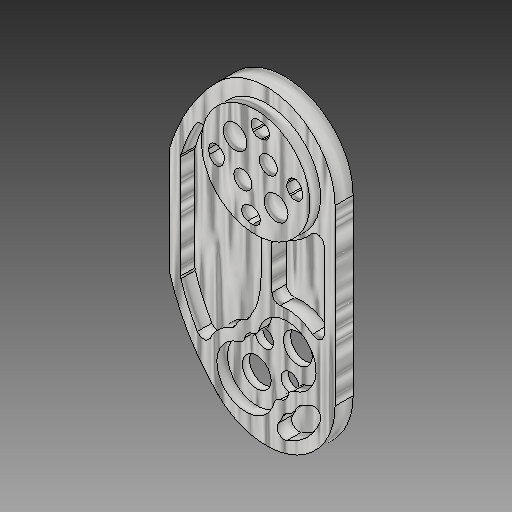
# Autodesk Inventor part: 新型３クランク
Saved by Autodesk Inventor 2019 (Build 230136000, 136)
## iProperties
Created: 2019-04-13
Part Number: 新型３クランク
Material: アルミニウム 7075
Document SubType Name: Modeling
Designer: tanjihayato
Density: 2.81 g/cm^3
Appearance: サテン - ブラシ仕上げ 重厚
Mass: 3.99356 g
Surface Area: 24.6385 cm^2
Volume: 1.42119 cm^3
Author: tanjihayato
Autodesk Inventor part; units mm, degrees
ref_plane "YZ Plane" through (0, 0, 0) normal (1, 0, 0) x (0, 1, 0)
ref_plane "XZ Plane" through (0, 0, 0) normal (0, 1, 0) x (-1, 0, 0)
ref_plane "XY Plane" through (0, 0, 0) normal (0, 0, 1) x (1, 0, 0)
sketch "スケッチ1" plane through (0, 0, 0) normal (0, 0, 1) x (1, 0, 0)
  circle A0 centre (-9.17471, -9.17471) radius 2
  circle A1 centre (-14.86692, -14.86692) radius 2
  circle A2 centre (-13.788582, -10.253048) radius 1.25
  circle A3 centre (-10.253048, -13.788582) radius 1.25
  arc A4 (-8.249894, -13.092023) -> (-9.012536, -13.942297) centre (-8.020125, -14.065269) ccw
  arc A5 (-10.099334, -15.029095) -> (-9.012536, -13.942297) centre (-10.253048, -13.788582) ccw
  arc A6 (-10.099334, -15.029095) -> (-10.949607, -15.791737) centre (-9.976362, -16.021505) ccw
  arc A7 (-15.791737, -10.949607) -> (-10.949607, -15.791737) centre (-14.86692, -14.86692) ccw
  arc A8 (-15.791737, -10.949607) -> (-15.029095, -10.099334) centre (-16.021505, -9.976362) ccw
  arc A9 (-13.942297, -9.012536) -> (-15.029095, -10.099334) centre (-13.788582, -10.253048) ccw
  arc A10 (-13.942297, -9.012536) -> (-13.092023, -8.249894) centre (-14.065269, -8.020125) ccw
  arc A11 (-8.249894, -13.092023) -> (-13.092023, -8.249894) centre (-9.17471, -9.17471) ccw
  circle A12 centre (-10.253048, 13.788582) radius 1.25
  circle A13 centre (-13.788582, 10.253048) radius 1.25
  circle A14 centre (-9.17471, 9.17471) radius 1.65
  circle A15 centre (-14.86692, 14.86692) radius 1.65
  line L0 (-14.86692, 14.86692) -> (-9.17471, 9.17471)
  line L1 (-10.253048, 13.788582) -> (-13.788582, 10.253048)
  line L2 (-9.17471, -9.17471) -> (-14.86692, -14.86692)
  line L3 (-13.788582, -10.253048) -> (-10.253048, -13.788582)
  circle A16 centre (-12.020815, 12.020815) radius 9.5
  circle A17 centre (-12.020815, -12.020815) radius 9.5
  arc A18 (-18.73833, 18.73833) -> (-18.73833, -18.73833) centre (0, 0) ccw
  arc A19 (-5.303301, -18.73833) -> (-5.303301, 18.73833) centre (-24.041631, 0) ccw
  point P0 (0, 0)
  dimension "d0" = 19
  dimension "d1" = 19
  dimension "d2" = 17
  dimension "d3" = 17
  dimension "d101" = 3.3
  dimension "d102" = 3.3
  constraints: 32 centre point, 24 point on circle, 8 end point, 4 tangent, 2 midpoint, 2 perpendicular, 1 coincident, 1 parallel, 2 other
  measures "d0" diameter of A16
  measures "d1" diameter of A17
  measures "d2" distance of A16.centre A18.centre
  measures "d3" distance of A16.centre A19.centre
  measures "d101" diameter of A14
  measures "d102" diameter of A15
sketch "スケッチ2" plane through (0, 0, 0) normal (0, 0, 1) x (1, 0, 0)
  circle A0 centre (-12.020815, 12.020815) radius 9.5
  arc A1 (-18.73833, 18.73833) -> (-18.73833, -18.73833) centre (0, 0) ccw
  circle A2 centre (-14.86692, 14.86692) radius 1.65
  circle A3 centre (-10.253048, 13.788582) radius 1.25
  circle A4 centre (-13.788582, 10.253048) radius 1.25
  circle A5 centre (-9.17471, 9.17471) radius 1.65
  circle A6 centre (-12.020815, -12.020815) radius 9.5
  arc A7 (-8.249894, -13.092023) -> (-13.092023, -8.249894) centre (-9.17471, -9.17471) ccw
  circle A8 centre (-9.17471, -9.17471) radius 2
  circle A9 centre (-13.788582, -10.253048) radius 1.25
  arc A10 (-13.942297, -9.012536) -> (-13.092023, -8.249894) centre (-14.065269, -8.020125) ccw
  arc A11 (-15.791737, -10.949607) -> (-15.029095, -10.099334) centre (-16.021505, -9.976362) ccw
  arc A12 (-15.791737, -10.949607) -> (-10.949607, -15.791737) centre (-14.86692, -14.86692) ccw
  circle A13 centre (-14.86692, -14.86692) radius 2
  circle A14 centre (-10.253048, -13.788582) radius 1.25
  arc A15 (-10.099334, -15.029095) -> (-10.949607, -15.791737) centre (-9.976362, -16.021505) ccw
  arc A16 (-10.099334, -15.029095) -> (-9.012536, -13.942297) centre (-10.253048, -13.788582) ccw
  arc A17 (-8.249894, -13.092023) -> (-9.012536, -13.942297) centre (-8.020125, -14.065269) ccw
  arc A18 (-7.629655, -14.427179) -> (-14.427179, -7.629655) centre (-9.17471, -9.17471) ccw
  arc A19 (-9.614451, -16.411976) -> (-7.629655, -14.427179) centre (-10.253048, -13.788582) ccw
  arc A20 (-16.411976, -9.614451) -> (-9.614451, -16.411976) centre (-14.86692, -14.86692) ccw
  arc A21 (-14.427179, -7.629655) -> (-16.411976, -9.614451) centre (-13.788582, -10.253048) ccw
  arc A22 (-11.918863, 15.976632) -> (-15.976632, 11.918863) centre (-14.86692, 14.86692) ccw
  arc A23 (-8.064999, 12.122767) -> (-11.918863, 15.976632) centre (-10.253048, 13.788582) ccw
  arc A24 (-15.976632, 11.918863) -> (-12.122767, 8.064999) centre (-13.788582, 10.253048) ccw
  arc A25 (-12.122767, 8.064999) -> (-8.064999, 12.122767) centre (-9.17471, 9.17471) ccw
  circle A26 centre (-12.020815, -12.020815) radius 8
  line L0 (-25.41653, 7.5) -> (-25.41653, -7.5)
  line L1 (-23.91653, 7.280082) -> (-23.91653, -7.280082)
  arc A27 (-21.491034, 12.772449) -> (-23.91653, 7.280082) centre (0, 0) ccw
  arc A28 (-23.91653, -7.280082) -> (-21.491034, -12.772449) centre (0, 0) ccw
  line L2 (-2.520815, 12.020815) -> (-2.520815, -12.020815)
  line L3 (-4.020815, 6.89734) -> (-4.020815, -6.89734)
  circle A29 centre (-12.020815, 12.020815) radius 7.5
  line L4 (-13.788582, -10.253048) -> (-4.046147, -19.995484) construction
  line L5 (-13.788582, 10.253048) -> (-4.086909, 19.954722) construction
  line L6 (-12.770815, 2.550467) -> (-12.770815, -2.550467)
  line L7 (-11.270815, 2.550467) -> (-11.270815, -2.550467)
  point P0 (0, 0)
  point P1 (-5.303301, -18.73833)
  point P2 (-5.303301, 18.73833)
  dimension "d5" = 1.45
  dimension "d7" = 1.45
  dimension "d12" = 1.5
  dimension "d13" = 1.5
  dimension "d14" = 1.5
  dimension "d15" = 1.5
  dimension "d19" = 1.5
  dimension "d20" = 15
  dimension "d21" = 1.5
  dimension "d22" = 1.5
  dimension "d23" = 1.5
  dimension "d24" = 1.5
  dimension "d29" = 15
  dimension "d33" = 1.5
  dimension "d34" = 0.75
  constraints: 22 point on circle, 16 end point, 12 centre point, 6 vertical, 2 point on line, 1 coincident, 1 parallel, 14 other
  measures "d5" radial gap between concentric circles of A16 A19
  measures "d7" radial gap between concentric circles of A9 A21
  measures "d12" radial gap between concentric circles of A3 A23
  measures "d13" radial gap between concentric circles of A2 A22
  measures "d14" radial gap between concentric circles of A24 A4
  measures "d15" radial gap between concentric circles of A25 A5
  measures "d20" distance of L0.start L0.end
  measures "d21" distance between parallel lines of L1 L0
  measures "d22" radial gap between concentric circles of A1 A27
  measures "d23" radial gap between concentric circles of A1 A28
  measures "d24" distance between parallel lines of L3 L2
  measures "d29" diameter of A29
  measures "d33" distance between parallel lines of L6 L7
  measures "d34" distance from line of point (-12.021, 12.021) L7
extrude "押し出し4" add sketch "スケッチ2" along normal blind 4 contours A23 A25 A24 A22 | A29
extrude "押し出し5" add sketch "スケッチ2" along normal blind 2.5 contours A0 | L2 A6 L3 A0 | A0 A27 L1 A28 A6 A1 L0 | A6 A20 A26 A18 | L7 A6 L6 A0 | A6 A18 A26 A20 | A20 A26 A12 | A18 A26 A7 | A20 A21 A18 A26 A7 A10 A9 A11 A12 | A26 A12 A15 A14 A17 A7 A18 A19 A20
extrude "押し出し6" add sketch "スケッチ2" along normal blind 1 contours A26 A12 | A12 A11 A9 A10 A7 A26 A17 A14 A15 | A26 A7
extrude "押し出し7" add sketch "スケッチ2" along normal blind 0.5 contours L3 A6 L7 A0 | A0 L6 A6 A28 L1 A27 | A26 A18 A21 A20 | A20 A21 A18 A26 A7 A10 A9 A11 A12 | A26 A12 A15 A14 A17 A7 A18 A19 A20 | A20 A19 A18 A26 | A12 A11 A9 A10 A7 A26 A17 A14 A15
extrude "押し出し8" add sketch "スケッチ2" along normal blind 1 contours A3 | A4
sketch "スケッチ3" plane through (-12.020815, 12.020815, 4) normal (0, 0, 1) x (1, 0, 0)
  circle A0 centre (2.846105, -2.846105) radius 1.65
  circle A1 centre (-2.846105, 2.846105) radius 1.65
  circle A2 centre (-1.767767, -1.767767) radius 1.25
  circle A3 centre (1.767767, 1.767767) radius 1.25
  circle A4 centre (0, 0) radius 7.5
  arc A5 (9.5, 0) -> (-6.717514, 6.717514) centre (0, 0) ccw
  circle A6 centre (-2.846105, 2.846105) radius 3.15
  circle A7 centre (2.846105, -2.846105) radius 3.15
  line L0 (-1.767767, -1.767767) -> (9.834677, 9.834677) construction
  arc A8 (-0.156324, 7.998473) -> (1.213798, 4.461392) centre (9.834677, 9.834677) ccw
  arc A9 (4.461392, 1.213798) -> (7.998473, -0.156324) centre (9.834677, 9.834677) ccw
  arc A10 (4.461392, 1.213798) -> (1.213798, 4.461392) centre (1.767767, 1.767767) ccw
  arc A11 (0.096916, 3.969104) -> (3.969104, 0.096916) centre (1.767767, 1.767767) ccw
  line L1 (9.5, -24.041631) -> (9.5, 0)
  arc A12 (-9.470219, 0.751633) -> (-0.75, -9.470348) centre (0, 0) ccw
  arc A13 (0.156324, -7.998473) -> (-1.213798, -4.461392) centre (-9.834677, -9.834677) ccw
  arc A14 (-4.461392, -1.213798) -> (-7.998473, 0.156324) centre (-9.834677, -9.834677) ccw
  arc A15 (-4.461392, -1.213798) -> (-1.213798, -4.461392) centre (-1.767767, -1.767767) ccw
  arc A16 (-0.096916, -3.969104) -> (-3.969104, -0.096916) centre (-1.767767, -1.767767) ccw
  circle A17 centre (0, 0) radius 8
  point P0 (12.020815, -12.020815)
  point P1 (-0.051687, 7.499822)
  point P2 (7.499822, -0.051687)
  point P3 (0.051687, -7.499822)
  point P4 (-7.499822, 0.051687)
  dimension "d46" = 1.5
  dimension "d47" = 1.5
  dimension "d53" = 16
  constraints: 32 point on circle, 11 centre point, 2 end point, 2 point on line, 1 coincident, 4 other
  measures "d46" radial gap between concentric circles of A1 A6
  measures "d47" radial gap between concentric circles of A0 A7
  measures "d53" diameter of A17
extrude "押し出し11" cut sketch "スケッチ3" against normal blind 3.5 contours A4 A9 A10 A8 | A4 A8 A17 A9 | A14 A15 A13 A4 | A4 A13 A17 A14
fillet "フィレット1" radius 1 26 edges at (-4.0223, 11.8645, 1.5) (-11.8645, 4.0223, 1.5) (-20.0193, 12.1771, 1.5) (-12.1771, 20.0193, 1.5) (-13.2346, 7.5594, 2.25) (-16.4822, 10.807, 2.25) (-10.807, 16.4822, 2.25) (-7.5594, 13.2346, 2.25) (-12.7708, 2.5505, 1.5) (-21.491, 12.7724, 1.5) (-21.491, -12.7724, 1.5) (-23.9165, 7.2801, 1.5) (-23.9165, -7.2801, 1.5) (-12.7708, -2.5505, 1.5) (-11.2708, -2.5505, 1.5) (-11.2708, 2.5505, 1.5) (-4.0208, 6.8973, 1.5) (-4.0208, -6.8973, 1.5) (-4.0684, -11.1498, 1.5) (-12.8918, -19.9733, 1.5) (-9.6145, -16.412, 1.5) (-7.6297, -14.4272, 1.5) (-14.4272, -7.6297, 1.5) (-16.412, -9.6145, 1.5) (-19.9733, -12.8918, 1.5) (-11.1498, -4.0684, 1.5)
sketch "スケッチ5" plane through (0, 0, 2.5) normal (0, 0, 1) x (1, 0, 0)
  arc A0 (-9.205581, -19.509103) -> (-4.532527, -14.83605) centre (-12.020815, -12.020815) ccw
  arc A1 (-10.377475, -18.000689) -> (-9.205581, -19.509103) centre (-9.557485, -18.573067) ccw
  arc A2 (-10.377475, -18.000689) -> (-9.760725, -16.842368) centre (-14.86692, -14.86692) ccw
  arc A3 (-9.213211, -16.280316) -> (-9.760725, -16.842368) centre (-8.828087, -17.203181) ccw
  arc A4 (-9.213211, -16.280316) -> (-7.761314, -14.828419) centre (-10.253048, -13.788582) ccw
  arc A5 (-7.199262, -14.280906) -> (-7.761314, -14.828419) centre (-6.83845, -15.213544) ccw
  arc A6 (-7.199262, -14.280906) -> (-6.040941, -13.664155) centre (-9.17471, -9.17471) ccw
  arc A7 (-4.532527, -14.83605) -> (-6.040941, -13.664155) centre (-5.468563, -14.484145) ccw
  arc A8 (-14.828419, -7.761314) -> (-14.280906, -7.199262) centre (-15.213544, -6.83845) ccw
  arc A9 (-14.828419, -7.761314) -> (-16.280316, -9.213211) centre (-13.788582, -10.253048) ccw
  arc A10 (-16.842368, -9.760725) -> (-16.280316, -9.213211) centre (-17.203181, -8.828087) ccw
  arc A11 (-16.842368, -9.760725) -> (-18.000689, -10.377475) centre (-14.86692, -14.86692) ccw
  arc A12 (-19.509103, -9.205581) -> (-18.000689, -10.377475) centre (-18.573067, -9.557485) ccw
  arc A13 (-14.83605, -4.532527) -> (-19.509103, -9.205581) centre (-12.020815, -12.020815) ccw
  arc A14 (-13.664155, -6.040941) -> (-14.83605, -4.532527) centre (-14.484145, -5.468563) ccw
  arc A15 (-13.664155, -6.040941) -> (-14.280906, -7.199262) centre (-9.17471, -9.17471) ccw
  arc A16 (-11.671378, 19.51267) -> (-19.51267, 11.671378) centre (-12.020815, 12.020815) ccw
  arc A17 (-10.697307, 19.910576) -> (-11.671378, 19.51267) centre (-10.862746, 18.924356) ccw
  arc A18 (-4.131054, 13.344324) -> (-10.697307, 19.910576) centre (-12.020815, 12.020815) ccw
  arc A19 (-4.52896, 12.370253) -> (-4.131054, 13.344324) centre (-5.117275, 13.178885) ccw
  arc A20 (-12.370253, 4.52896) -> (-4.52896, 12.370253) centre (-12.020815, 12.020815) ccw
  arc A21 (-13.344324, 4.131054) -> (-12.370253, 4.52896) centre (-13.178885, 5.117275) ccw
  arc A22 (-19.910576, 10.697307) -> (-13.344324, 4.131054) centre (-12.020815, 12.020815) ccw
  arc A23 (-19.51267, 11.671378) -> (-19.910576, 10.697307) centre (-18.924356, 10.862746) ccw
  arc A24 (-8.249894, -13.092023) -> (-13.092023, -8.249894) centre (-9.17471, -9.17471) ccw
  arc A25 (-8.249894, -13.092023) -> (-9.012536, -13.942297) centre (-8.020125, -14.065269) ccw
  arc A26 (-10.099334, -15.029095) -> (-9.012536, -13.942297) centre (-10.253048, -13.788582) ccw
  arc A27 (-10.099334, -15.029095) -> (-10.949607, -15.791737) centre (-9.976362, -16.021505) ccw
  arc A28 (-15.791737, -10.949607) -> (-10.949607, -15.791737) centre (-14.86692, -14.86692) ccw
  arc A29 (-15.791737, -10.949607) -> (-15.029095, -10.099334) centre (-16.021505, -9.976362) ccw
  arc A30 (-13.942297, -9.012536) -> (-15.029095, -10.099334) centre (-13.788582, -10.253048) ccw
  arc A31 (-13.942297, -9.012536) -> (-13.092023, -8.249894) centre (-14.065269, -8.020125) ccw
  line L0 (-12.770815, 1.667676) -> (-12.770815, -1.667676)
  arc A32 (-13.604149, -2.653689) -> (-12.770815, -1.667676) centre (-13.770815, -1.667676) ccw
  arc A33 (-13.604149, -2.653689) -> (-21.183069, -9.510218) centre (-12.020815, -12.020815) ccw
  arc A34 (-23.07033, -9.631192) -> (-21.183069, -9.510218) centre (-22.147517, -9.245944) ccw
  arc A35 (-23.871385, -7.426773) -> (-23.07033, -9.631192) centre (0, 0) ccw
  arc A36 (-23.91653, -7.129702) -> (-23.871385, -7.426773) centre (-22.91653, -7.129702) ccw
  line L1 (-23.91653, -7.129702) -> (-23.91653, 7.129702)
  arc A37 (-23.871385, 7.426773) -> (-23.91653, 7.129702) centre (-22.91653, 7.129702) ccw
  arc A38 (-23.07033, 9.631192) -> (-23.871385, 7.426773) centre (0, 0) ccw
  arc A39 (-21.183069, 9.510218) -> (-23.07033, 9.631192) centre (-22.147517, 9.245944) ccw
  arc A40 (-21.183069, 9.510218) -> (-13.604149, 2.653689) centre (-12.020815, 12.020815) ccw
  arc A41 (-12.770815, 1.667676) -> (-13.604149, 2.653689) centre (-13.770815, 1.667676) ccw
  line L2 (-4.020815, 4.194577) -> (-4.020815, -4.194577)
  arc A42 (-5.687482, -4.939933) -> (-4.020815, -4.194577) centre (-5.020815, -4.194577) ccw
  arc A43 (-5.687482, -4.939933) -> (-10.437482, -2.653689) centre (-12.020815, -12.020815) ccw
  arc A44 (-11.270815, -1.667676) -> (-10.437482, -2.653689) centre (-10.270815, -1.667676) ccw
  line L3 (-11.270815, -1.667676) -> (-11.270815, 1.667676)
  arc A45 (-10.437482, 2.653689) -> (-11.270815, 1.667676) centre (-10.270815, 1.667676) ccw
  arc A46 (-10.437482, 2.653689) -> (-5.687482, 4.939933) centre (-12.020815, 12.020815) ccw
  arc A47 (-4.020815, 4.194577) -> (-5.687482, 4.939933) centre (-5.020815, 4.194577) ccw
  arc A48 (-2.520815, 12.020815) -> (-18.73833, 18.73833) centre (-12.020815, 12.020815) ccw
  arc A49 (-18.73833, 18.73833) -> (-25.41653, 7.5) centre (0, 0) ccw
  line L4 (-25.41653, 7.5) -> (-25.41653, -7.5)
  arc A50 (-25.41653, -7.5) -> (-18.73833, -18.73833) centre (0, 0) ccw
  arc A51 (-18.73833, -18.73833) -> (-2.520815, -12.020815) centre (-12.020815, -12.020815) ccw
  line L5 (-2.520815, -12.020815) -> (-2.520815, 12.020815)
  arc A52 (-19.509103, -9.205581) -> (-18.000689, -10.377475) centre (-18.573067, -9.557485) ccw
  arc A53 (-18.000689, -10.377475) -> (-20.332512, -14.546097) centre (-14.86692, -14.86692) ccw
  arc A54 (-23.07033, -9.631192) -> (-20.332512, -14.546097) centre (0, 0) ccw
  arc A55 (-13.552192, -5.831142) -> (-12.770815, -1.667676) centre (-24.253751, -1.667676) ccw
  point P0 (0, 0)
  constraints: 7 point on circle, 3 centre point, 2 tangent
extrude "押し出し12" cut sketch "スケッチ5" against normal blind 2 contours A14 A13 A12 A53 A54 A34 A33 A32 A55
fillet "フィレット2" radius 1 1 edges at (-20.3325, -14.5461, 1.5)
sketch "スケッチ6" plane through (0, 0, 2.5) normal (0, 0, 1) x (1, 0, 0)
  arc A0 (-2.520815, 12.020815) -> (-18.73833, 18.73833) centre (-12.020815, 12.020815) ccw
  arc A1 (-18.73833, 18.73833) -> (-25.41653, 7.5) centre (0, 0) ccw
  line L0 (-25.41653, 7.5) -> (-25.41653, -7.5)
  arc A2 (-25.41653, -7.5) -> (-18.73833, -18.73833) centre (0, 0) ccw
  arc A3 (-18.73833, -18.73833) -> (-2.520815, -12.020815) centre (-12.020815, -12.020815) ccw
  line L1 (-2.520815, -12.020815) -> (-2.520815, 12.020815)
  line L2 (-4.020815, 4.194577) -> (-4.020815, -4.194577)
  arc A4 (-5.687482, -4.939933) -> (-4.020815, -4.194577) centre (-5.020815, -4.194577) ccw
  arc A5 (-5.687482, -4.939933) -> (-10.437482, -2.653689) centre (-12.020815, -12.020815) ccw
  arc A6 (-11.270815, -1.667676) -> (-10.437482, -2.653689) centre (-10.270815, -1.667676) ccw
  line L3 (-11.270815, -1.667676) -> (-11.270815, 1.667676)
  arc A7 (-10.437482, 2.653689) -> (-11.270815, 1.667676) centre (-10.270815, 1.667676) ccw
  arc A8 (-10.437482, 2.653689) -> (-5.687482, 4.939933) centre (-12.020815, 12.020815) ccw
  arc A9 (-4.020815, 4.194577) -> (-5.687482, 4.939933) centre (-5.020815, 4.194577) ccw
  arc A10 (-8.249894, -13.092023) -> (-13.092023, -8.249894) centre (-9.17471, -9.17471) ccw
  arc A11 (-8.249894, -13.092023) -> (-9.012536, -13.942297) centre (-8.020125, -14.065269) ccw
  arc A12 (-10.099334, -15.029095) -> (-9.012536, -13.942297) centre (-10.253048, -13.788582) ccw
  arc A13 (-10.099334, -15.029095) -> (-10.949607, -15.791737) centre (-9.976362, -16.021505) ccw
  arc A14 (-15.791737, -10.949607) -> (-10.949607, -15.791737) centre (-14.86692, -14.86692) ccw
  arc A15 (-15.791737, -10.949607) -> (-15.029095, -10.099334) centre (-16.021505, -9.976362) ccw
  arc A16 (-13.942297, -9.012536) -> (-15.029095, -10.099334) centre (-13.788582, -10.253048) ccw
  arc A17 (-13.942297, -9.012536) -> (-13.092023, -8.249894) centre (-14.065269, -8.020125) ccw
  arc A18 (-19.910576, 10.697307) -> (-13.344324, 4.131054) centre (-12.020815, 12.020815) ccw
  arc A19 (-19.51267, 11.671378) -> (-19.910576, 10.697307) centre (-18.924356, 10.862746) ccw
  arc A20 (-11.671378, 19.51267) -> (-19.51267, 11.671378) centre (-12.020815, 12.020815) ccw
  arc A21 (-10.697307, 19.910576) -> (-11.671378, 19.51267) centre (-10.862746, 18.924356) ccw
  arc A22 (-4.131054, 13.344324) -> (-10.697307, 19.910576) centre (-12.020815, 12.020815) ccw
  arc A23 (-4.52896, 12.370253) -> (-4.131054, 13.344324) centre (-5.117275, 13.178885) ccw
  arc A24 (-12.370253, 4.52896) -> (-4.52896, 12.370253) centre (-12.020815, 12.020815) ccw
  arc A25 (-13.344324, 4.131054) -> (-12.370253, 4.52896) centre (-13.178885, 5.117275) ccw
  arc A26 (-13.552192, -5.831142) -> (-12.770815, -1.667676) centre (-24.253751, -1.667676) ccw
  arc A27 (-13.664155, -6.040941) -> (-13.552192, -5.831142) centre (-14.484145, -5.468563) ccw
  arc A28 (-13.664155, -6.040941) -> (-14.280906, -7.199262) centre (-9.17471, -9.17471) ccw
  arc A29 (-14.828419, -7.761314) -> (-14.280906, -7.199262) centre (-15.213544, -6.83845) ccw
  arc A30 (-14.828419, -7.761314) -> (-16.280316, -9.213211) centre (-13.788582, -10.253048) ccw
  arc A31 (-16.842368, -9.760725) -> (-16.280316, -9.213211) centre (-17.203181, -8.828087) ccw
  arc A32 (-16.842368, -9.760725) -> (-19.818975, -12.531802) centre (-14.86692, -14.86692) ccw
  arc A33 (-21.586938, -12.609684) -> (-19.818975, -12.531802) centre (-20.72346, -12.105297) ccw
  arc A34 (-23.871385, -7.426773) -> (-21.586938, -12.609684) centre (0, 0) ccw
  arc A35 (-23.91653, -7.129702) -> (-23.871385, -7.426773) centre (-22.91653, -7.129702) ccw
  line L4 (-23.91653, -7.129702) -> (-23.91653, 7.129702)
  arc A36 (-23.871385, 7.426773) -> (-23.91653, 7.129702) centre (-22.91653, 7.129702) ccw
  arc A37 (-23.07033, 9.631192) -> (-23.871385, 7.426773) centre (0, 0) ccw
  arc A38 (-21.183069, 9.510218) -> (-23.07033, 9.631192) centre (-22.147517, 9.245944) ccw
  arc A39 (-21.183069, 9.510218) -> (-13.604149, 2.653689) centre (-12.020815, 12.020815) ccw
  arc A40 (-12.770815, 1.667676) -> (-13.604149, 2.653689) centre (-13.770815, 1.667676) ccw
  line L5 (-12.770815, 1.667676) -> (-12.770815, -1.667676)
  arc A41 (-9.205581, -19.509103) -> (-4.532527, -14.83605) centre (-12.020815, -12.020815) ccw
  arc A42 (-10.377475, -18.000689) -> (-9.205581, -19.509103) centre (-9.557485, -18.573067) ccw
  arc A43 (-10.377475, -18.000689) -> (-9.760725, -16.842368) centre (-14.86692, -14.86692) ccw
  arc A44 (-9.213211, -16.280316) -> (-9.760725, -16.842368) centre (-8.828087, -17.203181) ccw
  arc A45 (-9.213211, -16.280316) -> (-7.761314, -14.828419) centre (-10.253048, -13.788582) ccw
  arc A46 (-7.199262, -14.280906) -> (-7.761314, -14.828419) centre (-6.83845, -15.213544) ccw
  arc A47 (-7.199262, -14.280906) -> (-6.040941, -13.664155) centre (-9.17471, -9.17471) ccw
  arc A48 (-4.532527, -14.83605) -> (-6.040941, -13.664155) centre (-5.468563, -14.484145) ccw
  arc A49 (-5.662343, -4.974841) -> (-11.270815, -4.116848) centre (-9.17471, -9.17471) ccw
  line L6 (-11.270815, -1.667676) -> (-11.270815, -4.116848)
  arc A50 (-5.662343, -4.974841) -> (-4.020815, -4.207742) centre (-5.020815, -4.207742) ccw
  line L7 (-4.020815, 4.194577) -> (-4.020815, -4.194577)
  line L8 (-4.020815, -4.194577) -> (-4.020815, -4.207742)
  point P0 (0, 0)
  dimension "d60" = 2
  dimension "d61" = 1.45
  constraints: 4 end point, 4 point on circle, 2 centre point, 2 tangent, 2 vertical
  measures "d60" diameter of A50
  measures "d61" radial gap between concentric circles of A49 A10
extrude "押し出し13" cut sketch "スケッチ6" against normal blind 2 contours A50 A49 L6 A6 A5 A4
fillet "フィレット3" radius 1 1 edges at (-11.2708, -4.1168, 1.5)
sketch "スケッチ7" plane through (0, 0, 4) normal (0, 0, 1) x (1, 0, 0)
  arc A0 (-12.231485, 5.437326) -> (-12.896473, 6.974428) centre (-21.855492, 2.186138) ccw
  arc A1 (-12.370253, 4.52896) -> (-12.231485, 5.437326) centre (-13.178885, 5.117275) ccw
  arc A2 (-12.370253, 4.52896) -> (-4.52896, 12.370253) centre (-12.020815, 12.020815) ccw
  arc A3 (-5.437326, 12.231485) -> (-4.52896, 12.370253) centre (-5.117275, 13.178885) ccw
  arc A4 (-6.974428, 12.896473) -> (-5.437326, 12.231485) centre (-2.186138, 21.855492) ccw
  arc A5 (-7.503058, 13.781123) -> (-6.974428, 12.896473) centre (-6.503062, 13.778411) ccw
  arc A6 (-7.503058, 13.781123) -> (-10.260507, 16.538572) centre (-10.253048, 13.788582) ccw
  arc A7 (-11.145157, 17.067203) -> (-10.260507, 16.538572) centre (-10.26322, 17.538568) ccw
  arc A8 (-11.810146, 18.604305) -> (-11.145157, 17.067203) centre (-2.186138, 21.855492) ccw
  arc A9 (-11.671378, 19.51267) -> (-11.810146, 18.604305) centre (-10.862746, 18.924356) ccw
  arc A10 (-11.671378, 19.51267) -> (-19.51267, 11.671378) centre (-12.020815, 12.020815) ccw
  arc A11 (-18.604305, 11.810146) -> (-19.51267, 11.671378) centre (-18.924356, 10.862746) ccw
  arc A12 (-17.067203, 11.145157) -> (-18.604305, 11.810146) centre (-21.855492, 2.186138) ccw
  arc A13 (-16.538572, 10.260507) -> (-17.067203, 11.145157) centre (-17.538568, 10.26322) ccw
  arc A14 (-16.538572, 10.260507) -> (-13.781123, 7.503058) centre (-13.788582, 10.253048) ccw
  arc A15 (-12.896473, 6.974428) -> (-13.781123, 7.503058) centre (-13.778411, 6.503062) ccw
  circle A16 centre (-9.17471, 9.17471) radius 1.65
  circle A17 centre (-14.86692, 14.86692) radius 1.65
  circle A18 centre (-13.788582, 10.253048) radius 1.25
  circle A19 centre (-10.253048, 13.788582) radius 1.25
  circle A20 centre (-12.020815, 12.020815) radius 7.5
  point P0 (0, 0)
  constraints: 1 centre point, 1 coincident, 1 concentric
extrude "押し出し14" add sketch "スケッチ7" against normal blind 4 contours A1 A20 A11 A12 A13 A14 A15 A0 | A3 A4 A5 A6 A7 A8 A9 A20
sketch "スケッチ8" plane through (0, 0, 2.5) normal (0, 0, 1) x (1, 0, 0)
  line L0 (-11.270815, -2.793161) -> (-11.270815, 1.667676)
  arc A0 (-10.437482, 2.653689) -> (-11.270815, 1.667676) centre (-10.270815, 1.667676) ccw
  arc A1 (-10.437482, 2.653689) -> (-5.687482, 4.939933) centre (-12.020815, 12.020815) ccw
  arc A2 (-4.020815, 4.194577) -> (-5.687482, 4.939933) centre (-5.020815, 4.194577) ccw
  line L1 (-4.020815, 4.194577) -> (-4.020815, -4.207742)
  arc A3 (-5.662343, -4.974841) -> (-4.020815, -4.207742) centre (-5.020815, -4.207742) ccw
  arc A4 (-5.662343, -4.974841) -> (-10.101533, -3.778728) centre (-9.17471, -9.17471) ccw
  arc A5 (-11.270815, -2.793161) -> (-10.101533, -3.778728) centre (-10.270815, -2.793161) ccw
  arc A6 (-2.520815, 12.020815) -> (-18.73833, 18.73833) centre (-12.020815, 12.020815) ccw
  arc A7 (-18.73833, 18.73833) -> (-25.41653, 7.5) centre (0, 0) ccw
  line L2 (-25.41653, 7.5) -> (-25.41653, -7.5)
  arc A8 (-25.41653, -7.5) -> (-18.73833, -18.73833) centre (0, 0) ccw
  arc A9 (-18.73833, -18.73833) -> (-2.520815, -12.020815) centre (-12.020815, -12.020815) ccw
  line L3 (-2.520815, -12.020815) -> (-2.520815, 12.020815)
  arc A10 (-8.249894, -13.092023) -> (-13.092023, -8.249894) centre (-9.17471, -9.17471) ccw
  arc A11 (-8.249894, -13.092023) -> (-9.012536, -13.942297) centre (-8.020125, -14.065269) ccw
  arc A12 (-10.099334, -15.029095) -> (-9.012536, -13.942297) centre (-10.253048, -13.788582) ccw
  arc A13 (-10.099334, -15.029095) -> (-10.949607, -15.791737) centre (-9.976362, -16.021505) ccw
  arc A14 (-15.791737, -10.949607) -> (-10.949607, -15.791737) centre (-14.86692, -14.86692) ccw
  arc A15 (-15.791737, -10.949607) -> (-15.029095, -10.099334) centre (-16.021505, -9.976362) ccw
  arc A16 (-13.942297, -9.012536) -> (-15.029095, -10.099334) centre (-13.788582, -10.253048) ccw
  arc A17 (-13.942297, -9.012536) -> (-13.092023, -8.249894) centre (-14.065269, -8.020125) ccw
  arc A18 (-19.910576, 10.697307) -> (-13.344324, 4.131054) centre (-12.020815, 12.020815) ccw
  arc A19 (-19.51267, 11.671378) -> (-19.910576, 10.697307) centre (-18.924356, 10.862746) ccw
  arc A20 (-11.671378, 19.51267) -> (-19.51267, 11.671378) centre (-12.020815, 12.020815) ccw
  arc A21 (-10.697307, 19.910576) -> (-11.671378, 19.51267) centre (-10.862746, 18.924356) ccw
  arc A22 (-4.131054, 13.344324) -> (-10.697307, 19.910576) centre (-12.020815, 12.020815) ccw
  arc A23 (-4.52896, 12.370253) -> (-4.131054, 13.344324) centre (-5.117275, 13.178885) ccw
  arc A24 (-12.370253, 4.52896) -> (-4.52896, 12.370253) centre (-12.020815, 12.020815) ccw
  arc A25 (-13.344324, 4.131054) -> (-12.370253, 4.52896) centre (-13.178885, 5.117275) ccw
  arc A26 (-13.552192, -5.831142) -> (-12.770815, -1.667676) centre (-24.253751, -1.667676) ccw
  arc A27 (-13.664155, -6.040941) -> (-13.552192, -5.831142) centre (-14.484145, -5.468563) ccw
  arc A28 (-13.664155, -6.040941) -> (-14.280906, -7.199262) centre (-9.17471, -9.17471) ccw
  arc A29 (-14.828419, -7.761314) -> (-14.280906, -7.199262) centre (-15.213544, -6.83845) ccw
  arc A30 (-14.828419, -7.761314) -> (-16.280316, -9.213211) centre (-13.788582, -10.253048) ccw
  arc A31 (-16.842368, -9.760725) -> (-16.280316, -9.213211) centre (-17.203181, -8.828087) ccw
  arc A32 (-16.842368, -9.760725) -> (-19.818975, -12.531802) centre (-14.86692, -14.86692) ccw
  arc A33 (-21.586938, -12.609684) -> (-19.818975, -12.531802) centre (-20.72346, -12.105297) ccw
  arc A34 (-23.871385, -7.426773) -> (-21.586938, -12.609684) centre (0, 0) ccw
  arc A35 (-23.91653, -7.129702) -> (-23.871385, -7.426773) centre (-22.91653, -7.129702) ccw
  line L4 (-23.91653, -7.129702) -> (-23.91653, 7.129702)
  arc A36 (-23.871385, 7.426773) -> (-23.91653, 7.129702) centre (-22.91653, 7.129702) ccw
  arc A37 (-23.07033, 9.631192) -> (-23.871385, 7.426773) centre (0, 0) ccw
  arc A38 (-21.183069, 9.510218) -> (-23.07033, 9.631192) centre (-22.147517, 9.245944) ccw
  arc A39 (-21.183069, 9.510218) -> (-13.604149, 2.653689) centre (-12.020815, 12.020815) ccw
  arc A40 (-12.770815, 1.667676) -> (-13.604149, 2.653689) centre (-13.770815, 1.667676) ccw
  line L5 (-12.770815, 1.667676) -> (-12.770815, -1.667676)
  arc A41 (-9.205581, -19.509103) -> (-4.532527, -14.83605) centre (-12.020815, -12.020815) ccw
  arc A42 (-10.377475, -18.000689) -> (-9.205581, -19.509103) centre (-9.557485, -18.573067) ccw
  arc A43 (-10.377475, -18.000689) -> (-9.760725, -16.842368) centre (-14.86692, -14.86692) ccw
  arc A44 (-9.213211, -16.280316) -> (-9.760725, -16.842368) centre (-8.828087, -17.203181) ccw
  arc A45 (-9.213211, -16.280316) -> (-7.761314, -14.828419) centre (-10.253048, -13.788582) ccw
  arc A46 (-7.199262, -14.280906) -> (-7.761314, -14.828419) centre (-6.83845, -15.213544) ccw
  arc A47 (-7.199262, -14.280906) -> (-6.040941, -13.664155) centre (-9.17471, -9.17471) ccw
  arc A48 (-4.532527, -14.83605) -> (-6.040941, -13.664155) centre (-5.468563, -14.484145) ccw
  arc A49 (-19.51267, 11.671378) -> (-12.370253, 4.52896) centre (-12.020815, 12.020815) ccw
  arc A50 (-19.51267, 11.671378) -> (-19.910576, 10.697307) centre (-18.924356, 10.862746) ccw
  arc A51 (-19.910576, 10.697307) -> (-13.344324, 4.131054) centre (-12.020815, 12.020815) ccw
  arc A52 (-13.344324, 4.131054) -> (-12.370253, 4.52896) centre (-13.178885, 5.117275) ccw
  arc A53 (-4.52896, 12.370253) -> (-11.671378, 19.51267) centre (-12.020815, 12.020815) ccw
  arc A54 (-4.52896, 12.370253) -> (-4.131054, 13.344324) centre (-5.117275, 13.178885) ccw
  arc A55 (-4.131054, 13.344324) -> (-10.697307, 19.910576) centre (-12.020815, 12.020815) ccw
  arc A56 (-10.697307, 19.910576) -> (-11.671378, 19.51267) centre (-10.862746, 18.924356) ccw
  point P0 (0, 0)
extrude "押し出し15" add sketch "スケッチ8" against normal blind 2.5 contours A19 A49 A25 A18 | A21 A22 A23 A53
sketch "スケッチ9" plane through (-12.020815, 12.020815, 4) normal (0, 0, 1) x (1, 0, 0)
  circle A0 centre (0, 0) radius 7.5
  circle A1 centre (2.846105, -2.846105) radius 1.65
  circle A2 centre (-2.846105, 2.846105) radius 1.65
  circle A3 centre (-1.767767, -1.767767) radius 1.25
  circle A4 centre (1.767767, 1.767767) radius 1.25
  arc A5 (6.407505, 1.092648) -> (4.447344, 1.149407) centre (5.421735, 0.924548) ccw
  arc A6 (1.149407, 4.447344) -> (1.092648, 6.407505) centre (0.924548, 5.421735) ccw
  arc A7 (-1.149407, -4.447344) -> (-1.092648, -6.407505) centre (-0.924548, -5.421735) ccw
  arc A8 (-6.407505, -1.092648) -> (-4.447344, -1.149407) centre (-5.421735, -0.924548) ccw
  arc A9 (0.101952, 3.955817) -> (-2.543794, 5.981565) centre (-2.846105, 2.846105) ccw
  arc A10 (-5.981565, 2.543794) -> (-3.955817, -0.101952) centre (-2.846105, 2.846105) ccw
  arc A11 (-0.101952, -3.955817) -> (2.543794, -5.981565) centre (2.846105, -2.846105) ccw
  arc A12 (5.981565, -2.543794) -> (3.955817, 0.101952) centre (2.846105, -2.846105) ccw
  arc A13 (3.955817, 0.101952) -> (4.447344, 1.149407) centre (1.767767, 1.767767) ccw
  arc A14 (1.149407, 4.447344) -> (0.101952, 3.955817) centre (1.767767, 1.767767) ccw
  arc A15 (5.981565, -2.543794) -> (6.407505, 1.092648) centre (0, 0) ccw
  arc A16 (1.092648, 6.407505) -> (-2.543794, 5.981565) centre (0, 0) ccw
  arc A17 (-5.981565, 2.543794) -> (-6.407505, -1.092648) centre (0, 0) ccw
  arc A18 (-1.092648, -6.407505) -> (2.543794, -5.981565) centre (0, 0) ccw
  arc A19 (-3.955817, -0.101952) -> (-4.447344, -1.149407) centre (-1.767767, -1.767767) ccw
  arc A20 (-1.149407, -4.447344) -> (-0.101952, -3.955817) centre (-1.767767, -1.767767) ccw
  point P0 (12.020815, -12.020815)
  dimension "d74" = 2
  dimension "d75" = 2
  dimension "d76" = 2
  dimension "d77" = 2
  dimension "d84" = 1
  dimension "d85" = 6.5
  dimension "d86" = 2.75
  dimension "d87" = 2.75
  dimension "d88" = 2.75
  dimension "d89" = 6.5
  dimension "d90" = 6.5
  dimension "d91" = 2.75
  dimension "d103" = 1.5
  dimension "d104" = 1.5
  dimension "d105" = 1.5
  dimension "d106" = 1.5
  constraints: 32 point on circle, 16 centre point, 8 tangent
  measures "d74" diameter of A5
  measures "d75" diameter of A6
  measures "d76" diameter of A7
  measures "d77" diameter of A8
  measures "d84" radial gap between concentric circles of A0 A17
  measures "d85" radius of A18
  measures "d86" radius of A20
  measures "d87" radius of A19
  measures "d88" radius of A14
  measures "d89" radius of A16
  measures "d90" radius of A15
  measures "d91" radius of A13
  measures "d103" radial gap between concentric circles of A12 A1
  measures "d104" radial gap between concentric circles of A11 A1
  measures "d105" radial gap between concentric circles of A2 A10
  measures "d106" radial gap between concentric circles of A9 A2
extrude "押し出し16" cut sketch "スケッチ9" against normal blind 4 contours A15 A12 A13 A5 | A14 A9 A16 A6 | A20 A11 A18 A7 | A17 A10 A19 A8
fillet "フィレット4" radius 1 8 edges at (-6.0393, 9.477, 2) (-8.065, 12.1228, 2) (-9.477, 6.0393, 2) (-12.1228, 8.065, 2) (-15.9766, 11.9189, 2) (-18.0024, 14.5646, 2) (-14.5646, 18.0024, 2) (-11.9189, 15.9766, 2)
sketch "スケッチ10" plane through (0, 0, 2.5) normal (0, 0, 1) x (1, 0, 0)
  line L0 (-11.270815, -2.793161) -> (-11.270815, 1.667676)
  arc A0 (-10.437482, 2.653689) -> (-11.270815, 1.667676) centre (-10.270815, 1.667676) ccw
  arc A1 (-10.437482, 2.653689) -> (-5.687482, 4.939933) centre (-12.020815, 12.020815) ccw
  arc A2 (-4.020815, 4.194577) -> (-5.687482, 4.939933) centre (-5.020815, 4.194577) ccw
  line L1 (-4.020815, 4.194577) -> (-4.020815, -4.207742)
  arc A3 (-5.662343, -4.974841) -> (-4.020815, -4.207742) centre (-5.020815, -4.207742) ccw
  arc A4 (-5.662343, -4.974841) -> (-10.101533, -3.778728) centre (-9.17471, -9.17471) ccw
  arc A5 (-11.270815, -2.793161) -> (-10.101533, -3.778728) centre (-10.270815, -2.793161) ccw
  arc A6 (-2.520815, 12.020815) -> (-18.73833, 18.73833) centre (-12.020815, 12.020815) ccw
  arc A7 (-18.73833, 18.73833) -> (-25.41653, 7.5) centre (0, 0) ccw
  line L2 (-25.41653, 7.5) -> (-25.41653, -7.5)
  arc A8 (-25.41653, -7.5) -> (-18.73833, -18.73833) centre (0, 0) ccw
  arc A9 (-18.73833, -18.73833) -> (-2.520815, -12.020815) centre (-12.020815, -12.020815) ccw
  line L3 (-2.520815, -12.020815) -> (-2.520815, 12.020815)
  arc A10 (-8.249894, -13.092023) -> (-13.092023, -8.249894) centre (-9.17471, -9.17471) ccw
  arc A11 (-8.249894, -13.092023) -> (-9.012536, -13.942297) centre (-8.020125, -14.065269) ccw
  arc A12 (-10.099334, -15.029095) -> (-9.012536, -13.942297) centre (-10.253048, -13.788582) ccw
  arc A13 (-10.099334, -15.029095) -> (-10.949607, -15.791737) centre (-9.976362, -16.021505) ccw
  arc A14 (-15.791737, -10.949607) -> (-10.949607, -15.791737) centre (-14.86692, -14.86692) ccw
  arc A15 (-15.791737, -10.949607) -> (-15.029095, -10.099334) centre (-16.021505, -9.976362) ccw
  arc A16 (-13.942297, -9.012536) -> (-15.029095, -10.099334) centre (-13.788582, -10.253048) ccw
  arc A17 (-13.942297, -9.012536) -> (-13.092023, -8.249894) centre (-14.065269, -8.020125) ccw
  circle A18 centre (-12.020815, 12.020815) radius 7.5
  arc A19 (-13.552192, -5.831142) -> (-12.770815, -1.667676) centre (-24.253751, -1.667676) ccw
  arc A20 (-13.664155, -6.040941) -> (-13.552192, -5.831142) centre (-14.484145, -5.468563) ccw
  arc A21 (-13.664155, -6.040941) -> (-14.280906, -7.199262) centre (-9.17471, -9.17471) ccw
  arc A22 (-14.828419, -7.761314) -> (-14.280906, -7.199262) centre (-15.213544, -6.83845) ccw
  arc A23 (-14.828419, -7.761314) -> (-16.280316, -9.213211) centre (-13.788582, -10.253048) ccw
  arc A24 (-16.842368, -9.760725) -> (-16.280316, -9.213211) centre (-17.203181, -8.828087) ccw
  arc A25 (-16.842368, -9.760725) -> (-19.818975, -12.531802) centre (-14.86692, -14.86692) ccw
  arc A26 (-21.586938, -12.609684) -> (-19.818975, -12.531802) centre (-20.72346, -12.105297) ccw
  arc A27 (-23.871385, -7.426773) -> (-21.586938, -12.609684) centre (0, 0) ccw
  arc A28 (-23.91653, -7.129702) -> (-23.871385, -7.426773) centre (-22.91653, -7.129702) ccw
  line L4 (-23.91653, -7.129702) -> (-23.91653, 7.129702)
  arc A29 (-23.871385, 7.426773) -> (-23.91653, 7.129702) centre (-22.91653, 7.129702) ccw
  arc A30 (-23.07033, 9.631192) -> (-23.871385, 7.426773) centre (0, 0) ccw
  arc A31 (-21.183069, 9.510218) -> (-23.07033, 9.631192) centre (-22.147517, 9.245944) ccw
  arc A32 (-21.183069, 9.510218) -> (-13.604149, 2.653689) centre (-12.020815, 12.020815) ccw
  arc A33 (-12.770815, 1.667676) -> (-13.604149, 2.653689) centre (-13.770815, 1.667676) ccw
  line L5 (-12.770815, 1.667676) -> (-12.770815, -1.667676)
  arc A34 (-9.205581, -19.509103) -> (-4.532527, -14.83605) centre (-12.020815, -12.020815) ccw
  arc A35 (-10.377475, -18.000689) -> (-9.205581, -19.509103) centre (-9.557485, -18.573067) ccw
  arc A36 (-10.377475, -18.000689) -> (-9.760725, -16.842368) centre (-14.86692, -14.86692) ccw
  arc A37 (-9.213211, -16.280316) -> (-9.760725, -16.842368) centre (-8.828087, -17.203181) ccw
  arc A38 (-9.213211, -16.280316) -> (-7.761314, -14.828419) centre (-10.253048, -13.788582) ccw
  arc A39 (-7.199262, -14.280906) -> (-7.761314, -14.828419) centre (-6.83845, -15.213544) ccw
  arc A40 (-7.199262, -14.280906) -> (-6.040941, -13.664155) centre (-9.17471, -9.17471) ccw
  arc A41 (-4.532527, -14.83605) -> (-6.040941, -13.664155) centre (-5.468563, -14.484145) ccw
  circle A42 centre (-12.020815, 12.020815) radius 8
  line L6 (-4.020815, 4.194577) -> (-4.020815, 6.363961)
  line L7 (-11.270815, 1.667676) -> (-11.270815, 4.056049)
  arc A43 (-4.020815, 6.363961) -> (-5.798593, 6.9925) centre (-5.020815, 6.363961) ccw
  line L8 (-12.770815, 1.667676) -> (-12.770815, 4.056049)
  arc A44 (-21.886388, 12.082467) -> (-23.07033, 9.631192) centre (0, 0) ccw
  arc A45 (-20.012031, 11.646018) -> (-21.886388, 12.082467) centre (-21.010933, 11.599168) ccw
  point P0 (0, 0)
  dimension "d95" = 0.5
  dimension "d96" = 2
  dimension "d97" = 2
  constraints: 10 point on circle, 6 end point, 5 tangent, 4 centre point, 3 vertical, 1 concentric
  measures "d95" radial gap between concentric circles of A18 A42
  measures "d96" diameter of A43
  measures "d97" diameter of A45
extrude "押し出し17" cut sketch "スケッチ10" against normal blind 2 contours L7 A42 A43 L6 A2 A1 A0 | L8 A33 A32 A31 A44 A45 A42
fillet "フィレット5" radius 1 2 edges at (-12.7708, 4.056, 1.5) (-11.2708, 4.056, 1.5)
sketch "スケッチ11" plane through (-12.020815, 12.020815, 4) normal (0, 0, 1) x (1, 0, 0)
  arc A0 (-4.356451, -0.839749) -> (-4.447344, -1.149407) centre (-1.767767, -1.767767) ccw
  arc A1 (-6.407505, -1.092648) -> (-4.447344, -1.149407) centre (-5.421735, -0.924548) ccw
  arc A2 (-6.486534, -0.418182) -> (-6.407505, -1.092648) centre (0, 0) ccw
  arc A3 (-4.851858, 0.417226) -> (-6.486534, -0.418182) centre (-5.488606, -0.353847) ccw
  arc A4 (-4.851858, 0.417226) -> (-4.707023, 0.304553) centre (-2.846105, 2.846105) ccw
  arc A5 (-4.356451, -0.839749) -> (-4.707023, 0.304553) centre (-5.29779, -0.502289) ccw
  arc A6 (4.356451, 0.839749) -> (4.447344, 1.149407) centre (1.767767, 1.767767) ccw
  arc A7 (6.407505, 1.092648) -> (4.447344, 1.149407) centre (5.421735, 0.924548) ccw
  arc A8 (6.486534, 0.418182) -> (6.407505, 1.092648) centre (0, 0) ccw
  arc A9 (4.851858, -0.417226) -> (6.486534, 0.418182) centre (5.488606, 0.353847) ccw
  arc A10 (4.851858, -0.417226) -> (4.707023, -0.304553) centre (2.846105, -2.846105) ccw
  arc A11 (4.356451, 0.839749) -> (4.707023, -0.304553) centre (5.29779, 0.502289) ccw
  arc A12 (1.092648, 6.407505) -> (0.418182, 6.486534) centre (0, 0) ccw
  arc A13 (1.149407, 4.447344) -> (1.092648, 6.407505) centre (0.924548, 5.421735) ccw
  arc A14 (1.149407, 4.447344) -> (0.839749, 4.356451) centre (1.767767, 1.767767) ccw
  arc A15 (-0.304553, 4.707023) -> (0.839749, 4.356451) centre (0.502289, 5.29779) ccw
  arc A16 (-0.304553, 4.707023) -> (-0.417226, 4.851858) centre (-2.846105, 2.846105) ccw
  arc A17 (0.418182, 6.486534) -> (-0.417226, 4.851858) centre (0.353847, 5.488606) ccw
  arc A18 (-1.092648, -6.407505) -> (-0.418182, -6.486534) centre (0, 0) ccw
  arc A19 (-1.149407, -4.447344) -> (-1.092648, -6.407505) centre (-0.924548, -5.421735) ccw
  arc A20 (-1.149407, -4.447344) -> (-0.839749, -4.356451) centre (-1.767767, -1.767767) ccw
  arc A21 (0.304553, -4.707023) -> (-0.839749, -4.356451) centre (-0.502289, -5.29779) ccw
  arc A22 (0.304553, -4.707023) -> (0.417226, -4.851858) centre (2.846105, -2.846105) ccw
  arc A23 (-0.418182, -6.486534) -> (0.417226, -4.851858) centre (-0.353847, -5.488606) ccw
  circle A24 centre (0, 0) radius 7.5
  circle A25 centre (2.846105, -2.846105) radius 1.65
  circle A26 centre (-2.846105, 2.846105) radius 1.65
  circle A27 centre (-1.767767, -1.767767) radius 1.25
  circle A28 centre (1.767767, 1.767767) radius 1.25
  arc A29 (2.815234, -31.529918) -> (7.488288, -26.856865) centre (0, -24.041631) ccw
  arc A30 (1.64334, -30.021505) -> (2.815234, -31.529918) centre (2.46333, -30.593882) ccw
  arc A31 (1.64334, -30.021505) -> (2.26009, -28.863184) centre (-2.846105, -26.887735) ccw
  arc A32 (2.807604, -28.301132) -> (2.26009, -28.863184) centre (3.192729, -29.223996) ccw
  arc A33 (2.807604, -28.301132) -> (4.259501, -26.849234) centre (1.767767, -25.809398) ccw
  arc A34 (4.821553, -26.301721) -> (4.259501, -26.849234) centre (5.182366, -27.234359) ccw
  arc A35 (4.821553, -26.301721) -> (5.979874, -25.684971) centre (2.846105, -21.195526) ccw
  arc A36 (7.488288, -26.856865) -> (5.979874, -25.684971) centre (6.552252, -26.504961) ccw
  circle A37 centre (0, 0) radius 7.5
  arc A38 (3.770922, -25.112838) -> (-1.071208, -20.270709) centre (2.846105, -21.195526) ccw
  arc A39 (3.770922, -25.112838) -> (3.00828, -25.963112) centre (4.00069, -26.086084) ccw
  arc A40 (1.921482, -27.04991) -> (3.00828, -25.963112) centre (1.767767, -25.809398) ccw
  arc A41 (1.921482, -27.04991) -> (1.071208, -27.812552) centre (2.044453, -28.04232) ccw
  arc A42 (-3.770922, -22.970423) -> (1.071208, -27.812552) centre (-2.846105, -26.887735) ccw
  arc A43 (-3.770922, -22.970423) -> (-3.00828, -22.120149) centre (-4.00069, -21.997177) ccw
  arc A44 (-1.921482, -21.033351) -> (-3.00828, -22.120149) centre (-1.767767, -22.273864) ccw
  arc A45 (-1.921482, -21.033351) -> (-1.071208, -20.270709) centre (-2.044453, -20.040941) ccw
  arc A46 (9.5, 0) -> (-6.717514, 6.717514) centre (0, 0) ccw
  arc A47 (-6.717514, 6.717514) -> (-13.395715, -4.520815) centre (12.020815, -12.020815) ccw
  line L0 (-13.395715, -4.520815) -> (-13.395715, -19.520815)
  arc A48 (-13.395715, -19.520815) -> (-6.717514, -30.759145) centre (12.020815, -12.020815) ccw
  arc A49 (-6.717514, -30.759145) -> (9.5, -24.041631) centre (0, -24.041631) ccw
  line L1 (9.5, -24.041631) -> (9.5, 0)
  line L2 (0.75, -14.813976) -> (0.75, -8.828222)
  arc A50 (1.555556, -7.847308) -> (0.75, -8.828222) centre (1.75, -8.828222) ccw
  arc A51 (1.555556, -7.847308) -> (6.222222, -5.028315) centre (0, 0) ccw
  arc A52 (8, -5.656854) -> (6.222222, -5.028315) centre (7, -5.656854) ccw
  line L3 (8, -5.656854) -> (8, -16.228557)
  arc A53 (6.358472, -16.995656) -> (8, -16.228557) centre (7, -16.228557) ccw
  arc A54 (6.358472, -16.995656) -> (1.919283, -15.799543) centre (2.846105, -21.195526) ccw
  arc A55 (0.75, -14.813976) -> (1.919283, -15.799543) centre (1.75, -14.813976) ccw
  line L4 (-0.75, -8.828222) -> (-0.75, -13.688491)
  arc A56 (-1.531377, -17.851957) -> (-0.75, -13.688491) centre (-12.232936, -13.688491) ccw
  arc A57 (-1.64334, -18.061757) -> (-1.531377, -17.851957) centre (-2.46333, -17.489379) ccw
  arc A58 (-1.64334, -18.061757) -> (-2.26009, -19.220077) centre (2.846105, -21.195526) ccw
  arc A59 (-2.807604, -19.782129) -> (-2.26009, -19.220077) centre (-3.192729, -18.859265) ccw
  arc A60 (-2.807604, -19.782129) -> (-4.259501, -21.234027) centre (-1.767767, -22.273864) ccw
  arc A61 (-4.821553, -21.78154) -> (-4.259501, -21.234027) centre (-5.182366, -20.848902) ccw
  arc A62 (-4.821553, -21.78154) -> (-7.79816, -24.552617) centre (-2.846105, -26.887735) ccw
  arc A63 (-9.566122, -24.630499) -> (-7.79816, -24.552617) centre (-8.702645, -24.126112) ccw
  arc A64 (-11.85057, -19.447588) -> (-9.566122, -24.630499) centre (12.020815, -12.020815) ccw
  arc A65 (-11.895715, -19.150517) -> (-11.85057, -19.447588) centre (-10.895715, -19.150517) ccw
  line L5 (-11.895715, -19.150517) -> (-11.895715, -4.891113)
  arc A66 (-11.85057, -4.594042) -> (-11.895715, -4.891113) centre (-10.895715, -4.891113) ccw
  arc A67 (-9.865573, 0.061652) -> (-11.85057, -4.594042) centre (12.020815, -12.020815) ccw
  arc A68 (-7.991216, -0.374797) -> (-9.865573, 0.061652) centre (-8.990118, -0.421647) ccw
  arc A69 (-7.991216, -0.374797) -> (-1.555556, -7.847308) centre (0, 0) ccw
  arc A70 (-0.75, -8.828222) -> (-1.555556, -7.847308) centre (-1.75, -8.828222) ccw
  circle A71 centre (2.846105, -21.195526) radius 2
  arc A72 (3.00828, -25.963112) -> (1.921482, -27.04991) centre (1.767767, -25.809398) ccw
  arc A73 (-3.00828, -22.120149) -> (-1.921482, -21.033351) centre (-1.767767, -22.273864) ccw
  circle A74 centre (-2.846105, -26.887735) radius 2
  point P0 (12.020815, -12.020815)
